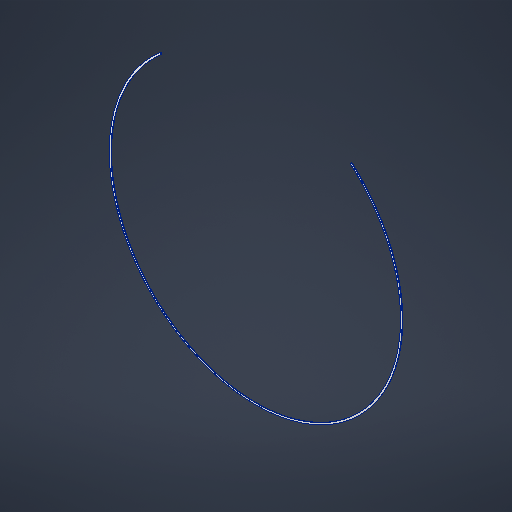
# Autodesk Inventor part: Support Ring
Saved by Autodesk Inventor 2026 (Build 300175000, 175)
## iProperties
Created: 2025-10-28
Part Number: Support Ring
Material: Aluminum 6061
Document SubType Name: Modeling
Designer: Brandon Portillo
Density: 2.7 g/cm^3
Appearance: Aluminum - Flat
Author: Brandon Portillo
Autodesk Inventor part; units mm, degrees
ref_plane "YZ Plane" through (0, 0, 0) normal (1, 0, 0) x (0, 1, 0)
ref_plane "XZ Plane" through (0, 0, 0) normal (0, 1, 0) x (-1, 0, 0)
ref_plane "XY Plane" through (0, 0, 0) normal (0, 0, 1) x (1, 0, 0)
sketch "Sketch1" plane through (0, 0, 0) normal (0, 0, 1) x (1, 0, 0)
  arc A0 (-1382.9892, 1613.371) -> (1382.9892, 1613.371) centre (0, 0) ccw
  arc A1 (-1370.2694, 1591.3396) -> (1370.2694, 1591.3396) centre (0, 0) ccw
  line L0 (-1370.2694, 1591.3396) -> (-1382.9892, 1613.371)
  line L1 (-1370.2694, 1591.3396) -> (-1344.8298, 1591.3396) construction
  line L2 (1370.2694, 1591.3396) -> (1382.9892, 1613.371)
  line L3 (1370.2694, 1591.3396) -> (1395.709, 1591.3396) construction
  dimension "d0" = 4250
  dimension "d1" = 4200
  dimension "d3" = 120
  dimension "d4" = 60
  constraints: 8 end point, 4 point on circle, 2 centre point, 2 coincident, 2 equal length, 2 horizontal
  measures "d0" diameter of A0
  measures "d1" diameter of A1
  measures "d3" angle of L1 L0
  measures "d4" angle of L3 L2
extrude "Extrusion1" add sketch "Sketch1" along normal blind 7
body "Solid1"
